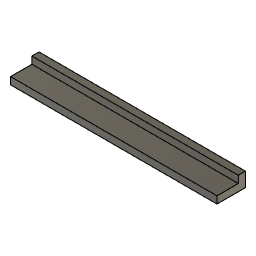
Attached v4 (Autodesk Fusion 360 design; units mm, degrees)
Autodesk Fusion 360 part; units mm, degrees
sketch "Esquisse1" plane through (0, 0, 0) normal (0, 0, 1) x (1, 0, 0)
  line L0 (0, 0) -> (58, 0)
  line L1 (58, 0) -> (58, 8)
  line L2 (58, 8) -> (0, 8)
  line L3 (0, 8) -> (0, 0)
  dimension "d1" = 58
  dimension "d2" = 8
  constraint horizontal L0
  constraint vertical L1
  constraint horizontal L2
  constraint vertical L3
  constraint coincident L0.start L3.end
  measures "d1" distance of L1.end L2.end
  measures "d2" distance of L0.end L1.end
extrude "Extrusion1" add sketch "Esquisse1" along normal blind 2
sketch "Esquisse2" plane through (0, 0, 2) normal (0, 0, 1) x (-1, 0, 0)
  line L0 (0, -8) -> (0, 0)
  line L1 (0, 0) -> (-58, 0)
  line L2 (-58, 0) -> (-58, -8)
  line L3 (-58, -8) -> (0, -8)
  line L4 (0, -8) -> (-58, -8)
  line L5 (-58, -8) -> (-58, -6)
  line L6 (-58, -6) -> (0, -6)
  line L7 (0, -6) -> (0, -8)
  dimension "d5" = 2
  constraint horizontal L4
  constraint vertical L5
  constraint horizontal L6
  constraint vertical L7
  constraint coincident L2 L5.end
  constraint coincident L0.start L3.end
  measures "d5" distance of L2.end L5.end
extrude "Extrusion2" add sketch "Esquisse2" along normal blind 2 contours L0 L2 L3 L4 L5 L6 L7
